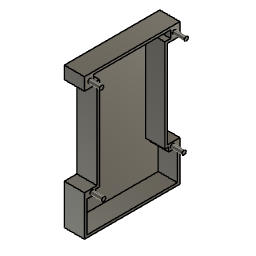
CAO Sablier Face Arrière avec fixations v3 (Autodesk Fusion 360 design; units mm, degrees)
Autodesk Fusion 360 part; units mm, degrees
note: some values were not read from the file. Set by a fixed rule: which face or edge a step refers to.
sketch "Esquisse1" plane through (0, 0, 0) normal (1, 0, 0) x (0, 1, 0)
  line L0 (0, 0) -> (114, 0)
  line L1 (114, 0) -> (114, 168)
  line L2 (114, 168) -> (0, 168)
  line L3 (0, 168) -> (0, 0)
  line L4 (0, 153) -> (15, 153)
  line L5 (15, 153) -> (15, 48)
  line L6 (15, 48) -> (0, 48)
  line L7 (0, 48) -> (0, 153)
  line L8 (57, 168) -> (57, 0)
  line L9 (114, 153) -> (99, 153)
  line L10 (99, 153) -> (99, 48)
  line L11 (99, 48) -> (114, 48)
  dimension "d1" = 114
  dimension "d2" = 168
  dimension "d3" = 15
  dimension "d4" = 48
  dimension "d5" = 15
  constraint horizontal L0
  constraint vertical L1
  constraint horizontal L2
  constraint vertical L3
  constraint coincident L0.start L3.end
  constraint horizontal L4
  constraint vertical L5
  constraint horizontal L6
  constraint vertical L7
  constraint coincident L3 L4.start
  constraint midpoint L2 L8.start
  constraint midpoint L0 L8.end
  constraint symmetric L4.start L8 L9.start
  constraint symmetric L4.end L8 L9.end
  constraint symmetric L5.end L8 L10.end
  constraint symmetric L6.end L8 L11.end
  measures "d1" distance of L1.end L2.end
  measures "d2" distance of L0.end L1.end
  measures "d3" distance of L2 L4
  measures "d4" distance of L0 L6
  measures "d5" distance of L5 L7
extrude "Extrusion1" add sketch "Esquisse1" along normal blind 20 contours L0 L2 L3 L4 L5 L6 L8
extrude "Extrusion2" add sketch "Esquisse1" along normal blind 20 contours L0 L1 L2 L8 L9 L10 L11
shell "Coque1" thickness 4 removed faces 1 at (20, 43, 118)
move_face "DécalerLesFaces1" offset 11 1 faces at (4, 44.3333, 119.3333)
extrude "Extrusion3" add 1 faces at (15, 44.3333, 119.3333) along direction (1, 0, 0) up to surface (5 mm away)
shell "Coque2" thickness 3 removed faces 1 at (20, 43, 118)
extrude "Extrusion4" cut 1 faces at (3, 44, 119) along direction (-1, 0, 0) blind 2
extrude "Extrusion5" add 1 faces at (0, 43, 118) along direction (-1, 0, 0) blind 5
extrude "Extrusion6" cut 1 faces at (1, 44, 119) along direction (-1, 0, 0) blind 5
extrude "Extrusion7" add 1 faces at (-4, 44, 119) along direction (1, 0, 0) blind 1
extrude "Extrusion8" cut 1 faces at (-5, 43, 118) along direction (1, 0, 0) blind 1
extrude "Extrusion9" add 1 faces at (4.6667, 111, 159) along direction (0, -1, 0) blind 10
extrude "Extrusion10" add 1 faces at (4.6667, 3, 162) along direction (0, 1, 0) blind 10
extrude "Extrusion11" add 1 faces at (12.3333, 8, 45) along direction (0, 0, -1) blind 5
sketch "Esquisse2" plane through (20, 0, 0) normal (1, 0, 0) x (0, 1, 0)
  line L0 (101, 156) -> (96, 156)
  line L1 (96, 156) -> (96, 45)
  line L2 (96, 45) -> (111, 45)
  line L3 (111, 45) -> (111, 3)
  line L4 (111, 3) -> (3, 3)
  line L5 (3, 3) -> (3, 40)
  line L6 (3, 40) -> (18, 40)
  line L7 (18, 40) -> (18, 156)
  line L8 (18, 156) -> (13, 156)
  line L9 (13, 156) -> (13, 165)
  line L10 (13, 165) -> (101, 165)
  line L11 (101, 165) -> (101, 156)
  line L12 (0, 168) -> (0, 153)
  line L13 (0, 153) -> (15, 153)
  line L14 (15, 153) -> (15, 48)
  line L15 (15, 48) -> (0, 48)
  line L16 (0, 48) -> (0, 0)
  line L17 (0, 0) -> (114, 0)
  line L18 (114, 0) -> (114, 48)
  line L19 (114, 48) -> (99, 48)
  line L20 (99, 48) -> (99, 153)
  line L21 (99, 153) -> (114, 153)
  line L22 (114, 153) -> (114, 168)
  line L23 (114, 168) -> (0, 168)
  line L24 (57, 168) -> (57, 0)
  circle A0 centre (6.5, 160.5) radius 2.45
  circle A1 centre (9, 44) radius 2.45
  circle A2 centre (107.5, 160.5) radius 2.45
  circle A3 centre (105, 44) radius 2.45
  line L25 (18, 45) -> (13.5, 45)
  line L26 (13.5, 45) -> (13.5, 40)
  line L27 (13.5, 40) -> (18, 40)
  line L28 (18, 40) -> (18, 45)
  line L29 (100.5, 45) -> (100.5, 40)
  line L30 (96, 45) -> (100.5, 45)
  line L31 (100.5, 40) -> (96, 40)
  line L32 (96, 40) -> (96, 45)
  dimension "d31" = 4.9
  dimension "d32" = 7.5
  dimension "d33" = 6.5
  dimension "d34" = 4.9
  dimension "d35" = 9
  dimension "d36" = 4
  dimension "d59" = 3
  dimension "d60" = 4.5
  constraint midpoint L23 L24.start
  constraint midpoint L17 L24.end
  constraint symmetric L24 A0 A2
  constraint symmetric L24 A1 A3
  constraint horizontal L25
  constraint vertical L26
  constraint horizontal L27
  constraint vertical L28
  constraint coincident L6 L26.end
  constraint coincident L7 L25.start
  constraint symmetric L24 L25.start L1.end
  constraint symmetric L24 L25.end L29.start
  constraint symmetric L24 L26.end L29.end
  constraint symmetric L24 L6.end L31.end
  measures "d31" diameter of A0
  measures "d32" distance of L13 A0.centre
  measures "d33" distance of L9 A0.centre
  measures "d34" diameter of A1
  measures "d35" distance of L16 A1.centre
  measures "d36" distance of L15 A1.centre
  measures "d59" distance of L15 L25
  measures "d60" distance of A1.centre L26
extrude "Extrusion12" add 1 faces at (12.3333, 101, 45) along direction (0, 0, -1) blind 5
extrude "Extrusion13" add sketch "Esquisse2" along normal blind 15 contours A1
extrude "Extrusion14" add sketch "Esquisse2" along normal blind 15 contours L2 A3 picked at (104.4042, 43.5271)
extrude "Extrusion15" add sketch "Esquisse2" along normal blind 15 contours L2 A3 picked at (105.5379, 45.488)
extrude "Extrusion16" add sketch "Esquisse2" along normal blind 15 contours A0
extrude "Extrusion17" cut 1 faces at (35, 7.1433, 159.3495) along direction (-1, 0, 0) blind 1
extrude "Extrusion18" add sketch "Esquisse2" along normal blind 14 contours A2
extrude "Extrusion19" cut 1 faces at (35, 8.8183, 44.7962) along direction (-1, 0, 0) blind 1
extrude "Extrusion20" cut 1 faces at (35, 104.3475, 42.6787) along direction (-1, 0, 0) blind 1
extrude "Extrusion21" cut 1 faces at (4.6667, 13, 162) along direction (0, -1, 0) blind 2
extrude "Extrusion22" cut 1 faces at (4.6667, 101, 159) along direction (0, 1, 0) blind 2
extrude "Extrusion23" cut sketch "Esquisse2" against normal blind 23 contours L6 L7 L25 L26 L27 L28
extrude "Extrusion24" cut sketch "Esquisse2" against normal blind 23 contours L2 L29 L30 L31 L32
